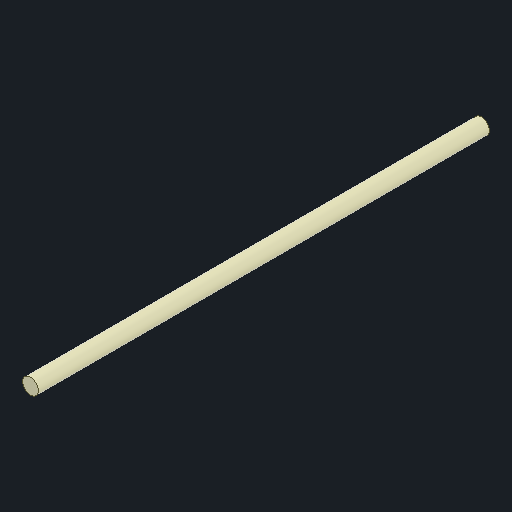
# Autodesk Inventor part: Type 1A 連接軸 1:9
Saved by Autodesk Inventor 2025.3 (Build 293356030, 356C)
## iProperties
Created: 2024-10-01
Part Number: Type 1A 連接軸 1:9
Material: 密度7850的鋼
Document SubType Name: Modeling
Designer: veter
Density: 7.84999 g/cm^3
Appearance: 平滑 - 暗灰色
Mass: 3273.2 g
Surface Area: 640.418 cm^2
Volume: 416.969 cm^3
Stock Number: 9
Author: veter
Autodesk Inventor part; units mm, degrees
ref_plane "YZ Plane" through (0, 0, 0) normal (1, 0, 0) x (0, 1, 0)
ref_plane "XZ Plane" through (0, 0, 0) normal (0, 1, 0) x (-1, 0, 0)
ref_plane "XY Plane" through (0, 0, 0) normal (0, 0, 1) x (1, 0, 0)
sketch "草圖1" plane through (0, 0, 0) normal (0, 0, 1) x (0, 1, 0)
  circle A0 centre (0, 0) radius 13.25
  dimension "d0" = 26.5
  constraints: 1 centre point, 1 coincident
  measures "d0" diameter of A0
extrude "擠出1" add sketch "草圖1" along normal mid plane 756
equation "\"d1\" = Width"
equation "\"Width\" = T1A_Joint_Width"
equation "\"T1A_Joint_Width\" = 756"
equation "\"T1A_R1\" = 585.5331"
equation "\"T1A_R3\" = 252.3048"
equation "\"T1A_R4\" = 320.6953"
equation "\"T1A_R5\" = 419.3047"
equation "\"T1A_R7\" = -221.7475"
equation "\"T1A_R8\" = 369.2781"
equation "\"T1A_R1_Width\" = 756"
equation "\"T1A_R2_Width\" = 756"
equation "\"T1A_R3_Width\" = 344"
equation "\"T1A_R4_Width\" = 756"
